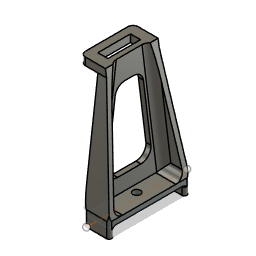
Deckbox_v2_Floor_Assembly (Autodesk Fusion 360 archive; units mm, degrees)
design "DC_DC_Clamp_2_0"
Autodesk Fusion 360 part; units mm, degrees
sketch "Skizze1" plane through (0, 0, 0) normal (0, 0, 1) x (1, 0, 0)
  line L0 (0, 0) -> (0, 46)
  line L1 (0, 46) -> (-7, 46)
  line L2 (-7, 46) -> (-7, 49)
  line L3 (-7, 49) -> (3, 49)
  line L4 (3, 49) -> (3, 2)
  line L5 (3, 2) -> (10, 2)
  line L6 (10, 2) -> (10, 0)
  line L7 (10, 0) -> (0, 0)
  line L8 (3, 49) -> (10, 2)
  dimension "d1" = 46
  dimension "d2" = 3
  dimension "d3" = 7
  dimension "d4" = 10
  dimension "d5" = 2
  dimension "d6" = 3
  constraint coincident L0.start L7.end
  constraint vertical L0
  constraint perpendicular L0 L1
  constraint perpendicular L1 L2
  constraint perpendicular L2 L3
  constraint perpendicular L3 L4
  constraint perpendicular L2 L5
  constraint perpendicular L5 L6
  constraint perpendicular L0 L7
  measures "d1" distance of L0.start L1
  measures "d2" distance of L1.end L2.end
  measures "d3" distance of L0.end L1.end
  measures "d4" distance of L6.end L0.start
  measures "d5" distance of L5 L7
  measures "d6" distance of L0 L4
extrude "Extrusion1" add sketch "Skizze1" along normal mid plane 32
sketch "Skizze2" plane through (0, 49, 0) normal (0, 1, 0) x (-1, 0, 0)
  line L0 (7, -16) -> (7, 16)
  line L1 (7, 16) -> (-3, 16)
  line L2 (-3, -16) -> (7, -16)
  line L3 (36, 0) -> (0, 0) construction
  line L4 (4, -6.5) -> (0, -6.5)
  line L5 (0, -6.5) -> (0, 6.5)
  line L6 (0, 6.5) -> (4, 6.5)
  line L7 (4, 6.5) -> (4, -6.5)
  line L8 (-3, 16) -> (-3, -16)
  dimension "d9" = 13
  dimension "d10" = 4
  constraint coincident L3.end origin
  constraint horizontal L3
  constraint horizontal L4
  constraint vertical L5
  constraint horizontal L6
  constraint vertical L7
  constraint symmetric L3 L4 L6
  constraint coincident L3.end L5
  measures "d9" distance of L4 L6
  measures "d10" distance of L4.start L4.end
extrude "Extrusion2" cut sketch "Skizze2" against normal through all contours L4 L5 L6 L7
sketch "Skizze3" plane through (0, 0, 0) normal (1, 0, 0) x (0, 0, -1)
  line L0 (10.5, 49) -> (-10.5, 49)
  line L1 (-10.5, 49) -> (-10.5, 46)
  line L2 (-10.5, 46) -> (10.5, 46) construction
  line L3 (10.5, 46) -> (10.5, 49)
  line L4 (0, 0) -> (0, 53) construction
  line L5 (16, 0) -> (-16, 0) construction
  line L6 (-16, 0) -> (-16, 2) construction
  line L7 (-16, 2) -> (16, 2) construction
  line L8 (16, 2) -> (16, 0) construction
  line L9 (16, 2) -> (10.5, 46)
  line L10 (-16, 2) -> (-10.5, 46)
  line L11 (16, 46) -> (-16, 46)
  line L12 (16, 49) -> (-16, 49)
  line L13 (16, 0) -> (-16, 0)
  line L14 (16, 0) -> (16, 46)
  line L15 (-16, 46) -> (-16, 0)
  line L16 (16, 2) -> (16, 50)
  line L17 (16, 50) -> (-16, 50)
  line L18 (-16, 50) -> (-16, 2)
  line L19 (0, 8) -> (9.2033, 8)
  line L20 (9.2033, 8) -> (5.2033, 40)
  line L21 (5.2033, 40) -> (0, 40)
  line L22 (-5.2033, 40) -> (0, 40)
  line L23 (-9.2033, 8) -> (-5.2033, 40)
  line L24 (0, 8) -> (-9.2033, 8)
  dimension "d12" = 2
  dimension "d13" = 21
  dimension "d14" = 50
  dimension "d23" = 6
  dimension "d24" = 6
  dimension "d25" = 6
  constraint horizontal L0
  constraint vertical L1
  constraint horizontal L2
  constraint vertical L3
  constraint coincident L4.start origin
  constraint perpendicular L0 L4
  constraint symmetric L1 L3 L4
  constraint horizontal L5
  constraint vertical L6
  constraint horizontal L7
  constraint vertical L8
  constraint collinear L2 L11
  constraint collinear L0 L12
  constraint collinear L5 L13
  constraint collinear L8 L14
  constraint collinear L6 L15
  constraint perpendicular L7 L16
  constraint perpendicular L16 L17
  constraint coincident L4 L19.start
  constraint perpendicular L4 L19
  constraint perpendicular L4 L21
  constraint coincident L4 L21.end
  constraint parallel L9 L20
  constraint symmetric L4 L19.start L24.start
  constraint symmetric L4 L19.end L23.start
  constraint symmetric L4 L20.end L22.start
  constraint symmetric L4 L21.end L22.end
  measures "d12" distance of L5 L7
  measures "d13" distance of L1 L3
  measures "d14" distance of L4.start L17
  measures "d23" distance of L7 L19
  measures "d24" distance of L9 L20
  measures "d25" distance of L2 L21
extrude "Extrusion3" cut sketch "Skizze3" along normal through all and the other way through all contours L3 L11 L12 L16 | L1 L11 L12 L18 | L9 L11 L14 L16 | L10 L11 L15 L18 | L19 L20 L21 L22 L23 L24
sketch "Skizze6" plane through (10, 0, 0) normal (1, 0, 0) x (0, 0, -1)
  line L0 (16, 2) -> (-16, 2)
  line L1 (-16, 2) -> (-16, 0)
  line L2 (-16, 0) -> (16, 0)
  line L3 (16, 0) -> (16, 2)
  line L4 (0, 2) -> (13.9844, 2)
  line L5 (13.9844, 2) -> (8.1094, 49)
  line L6 (8.1094, 49) -> (-0.0505, 49)
  line L7 (-0.0505, 61) -> (-0.0505, 49) construction
  line L8 (0, 2) -> (0, -14) construction
  line L9 (-10.5, 49) -> (10.5, 49)
  line L10 (16, 2) -> (10.5, 46)
  line L11 (-8.2104, 49) -> (-0.0505, 49)
  line L12 (-14.0854, 2) -> (-8.2104, 49)
  line L13 (-0.1009, 2) -> (-14.0854, 2)
  dimension "d20" = 2
  constraint coincident L0 L4.end
  constraint parallel L0 L6
  constraint vertical L7
  constraint coincident L0 L4.start
  constraint collinear L7 L8
  constraint collinear L6 L9
  constraint parallel L5 L10
  constraint coincident origin L8
  constraint symmetric L4.end L7 L12.start
  constraint symmetric L5.end L7 L11.start
  constraint symmetric L6.end L7 L11.end
  constraint symmetric L4.start L7 L13.start
  measures "d20" distance of L5 L10
extrude "Extrusion5" cut sketch "Skizze6" against normal blind 8 contours L0 L4 L5 L6 L9 L11 L12 L13
sketch "Skizze4" plane through (0, 0, 0) normal (0, 1, 0) x (1, 0, 0)
  line L0 (-10, 0) -> (15, 0) construction
  circle A0 centre (5, 0) radius 1.5
  dimension "d16" = 5
  dimension "d17" = 3
  constraint horizontal L0
  constraint coincident L0 A0.centre
  measures "d16" distance of origin A0.centre
  measures "d17" diameter of A0
extrude "Extrusion4" cut sketch "Skizze4" along normal through all
sketch "Skizze7" plane through (0, 0, 0) normal (0, -1, 0) x (1, 0, 0)
  circle A0 centre (5, 0) radius 1.5
  line L0 (10, -16) -> (10, 16)
  line L1 (10, 16) -> (0, 16)
  line L2 (0, 16) -> (0, -16)
  line L3 (0, -16) -> (10, -16)
  line L4 (5, -20) -> (5, 20) construction
  constraint perpendicular L1 L4
fillet "Abrundung1" radius 4 4 edges at (1, 8, -9.2033) (1, 8, 9.2033) (1, 40, -5.2033) (1, 40, 5.2033)
fillet "Abrundung2" radius 3 4 edges at (6, 2, 14.0854) (6, 2, -13.9844) (2, 25.5, 11.1479) (2, 25.5, -11.0469)
fillet "Abrundung3" radius 2 2 edges at (-7, 47.5, -10.5) (-7, 47.5, 10.5)
sketch "Skizze8" plane through (0, 0, 0) normal (0, -1, 0) x (1, 0, 0)
  line L0 (10, 16) -> (0, 16)
  line L1 (0, 16) -> (0, 14)
  line L2 (0, 14) -> (10, 14)
  line L3 (10, 14) -> (10, 16)
  line L4 (10, 16) -> (0, 16)
  line L5 (0, 0) -> (21, 0) construction
  line L6 (5, 0) -> (5, 31) construction
  line L7 (10, -16) -> (10, 16)
  line L8 (0, 16) -> (0, -16)
  line L9 (0, -14) -> (10, -14)
  line L10 (0, -16) -> (0, -14)
  line L11 (10, -16) -> (0, -16)
  line L12 (10, -14) -> (10, -16)
  dimension "d32" = 2
  dimension "d33" = 10
  constraint horizontal L0
  constraint vertical L1
  constraint horizontal L2
  constraint vertical L3
  constraint collinear L0 L4
  constraint coincident L5.start origin
  constraint horizontal L5
  constraint coincident L5 L6.start
  constraint perpendicular L2 L6
  constraint symmetric L1 L3 L6
  constraint symmetric L6 L7 L8
  constraint symmetric L0.start L5 L7.start
  constraint symmetric L0.end L5 L8.end
  constraint symmetric L1.end L5 L9.start
  constraint symmetric L2.end L5 L9.end
  measures "d32" distance of L0 L2
  measures "d33" distance of L1 L3
extrude "Extrusion6" add sketch "Skizze8" along normal blind 4 contours L0 L1 L2 L3 L4 L7 L8 | L7 L8 L9 L10 L11 L12
fillet "Abrundung4" radius 1 10 edges at (10, -2, 14) (10, -1, 16) (0, -1, 16) (0, -2, 14) (10, -2, -14) (0, -2, -14) (0, -1, -16) (10, -1, -16) (5, 0, 14) (5, 0, -14)

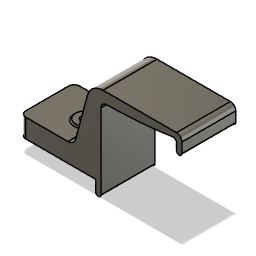
design "Pi_haken_2_0"
Autodesk Fusion 360 part; units mm, degrees
sketch "Skizze1" plane through (0, 0, 0) normal (0, 0, 1) x (1, 0, 0)
  line L0 (-85.7317, 64) -> (69.3607, 64) construction
  line L1 (2, 64) -> (2, 62) construction
  line L2 (2, 62) -> (-37, 62) construction
  arc A0 (3.9784, 62.0107) -> (29, 64) centre (2, 245.25) ccw
  line L3 (29, 64) -> (30, 63.25)
  line L4 (32, 63.25) -> (32, 66)
  line L5 (32, 66) -> (2.7668, 66)
  line L6 (-8, 43) -> (-28, 43)
  line L7 (-28, 43) -> (-28, 41)
  line L8 (2, 41) -> (2, 60.0108)
  line L9 (30, 63.25) -> (30, 59.25)
  line L10 (30, 59.25) -> (32, 59.25)
  line L11 (32, 59.25) -> (32, 63.25)
  line L12 (0, 41) -> (0, 31)
  line L13 (0, 31) -> (2, 31)
  line L14 (2, 31) -> (2, 41)
  line L15 (-95, 41) -> (0, 41) construction
  line L16 (2, 41) -> (26.9938, 41) construction
  line L17 (-28, 41) -> (0, 41)
  line L18 (-8, 43) -> (-3.0288, 61.5529)
  arc A1 (3.9784, 62.0107) -> (2, 60.0108) centre (4, 60.0108) ccw
  arc A2 (2.7668, 66) -> (-3.0288, 61.5529) centre (2.7668, 60) ccw
  line L19 (0, 81.6118) -> (0, 79.7535)
  line L20 (0, 79.7535) -> (0, 12.6342) construction
  point P0 (29, 64)
  dimension "d1" = 64
  dimension "d2" = 41
  dimension "d3" = 2
  dimension "d4" = 2
  dimension "d5" = 27
  dimension "d6" = 1
  dimension "d7" = 4
  dimension "d8" = 2
  dimension "d9" = 2
  dimension "d10" = 10
  dimension "d11" = 28
  dimension "d14" = 2
  dimension "d15" = 6
  dimension "d16" = 15
  dimension "d17" = 10
  dimension "d19" = 2
  constraint horizontal L0
  constraint horizontal L15
  constraint coincident L0 L1.start
  constraint perpendicular L0 L1
  constraint coincident L0 P0
  constraint perpendicular L1 L2
  constraint tangent L2 A0
  constraint coincident P0 A0.end
  constraint perpendicular L4 L5
  constraint coincident L7.end L15
  constraint perpendicular L7 L15
  constraint coincident L8.start L15
  constraint collinear L1 L8
  constraint perpendicular L9 L10
  constraint collinear L4 L11
  constraint vertical L12
  constraint horizontal L13
  constraint vertical L14
  constraint collinear L15 L16
  constraint perpendicular L12 L17
  constraint coincident L1.end L8
  constraint coincident L1.end A0
  constraint tangent L8 A1
  constraint tangent A0 A1
  constraint tangent L18 A2
  constraint tangent L5 A2
  constraint parallel L6 L15
  constraint horizontal L5
  constraint vertical L19
  constraint coincident origin L20
  constraint vertical L20
  constraint collinear L12 L20
  measures "d1" distance of origin L0
  measures "d2" distance of origin L15
  measures "d3" distance of origin L1
  measures "d4" distance of L1.start L1.end
  measures "d5" distance of L1 P0
  measures "d6" horizontal distance of P0 L3.end
  measures "d7" distance of L3.end L9.end
  measures "d8" distance of L9.end L10.end
  measures "d9" distance of P0 L5
  measures "d10" distance of L13 L16
  measures "d11" distance of L7.end L12.start
  measures "d14" radius of A1
  measures "d15" radius of A2
  measures "d16" angle of L8 L18
  measures "d17" distance of L6.start L8
  measures "d19" vertical distance of L6.end L12.start
extrude "Extrusion1" add sketch "Skizze1" along normal mid plane 20
sketch "Skizze2" plane through (0, 0, 0) normal (-1, 0, 0) x (0, 0, 1)
  line L0 (-10, 41) -> (-4.05, 41)
  line L1 (-4.05, 41) -> (-4.05, 36)
  line L2 (-4.05, 36) -> (-10, 36)
  line L3 (-10, 36) -> (-10, 41)
  line L4 (-10, 31) -> (-10, 41)
  line L5 (-10, 41) -> (10, 41)
  line L6 (0, 57.7062) -> (0, 0) construction
  line L7 (10, 36) -> (10, 41)
  line L8 (4.05, 36) -> (10, 36)
  line L9 (4.05, 41) -> (4.05, 36)
  line L10 (10, 41) -> (4.05, 41)
  dimension "d21" = 5.95
  dimension "d22" = 5
  constraint horizontal L0
  constraint vertical L1
  constraint horizontal L2
  constraint vertical L3
  constraint collinear L3 L4
  constraint collinear L0 L5
  constraint vertical L6
  constraint coincident L6.end origin
  constraint symmetric L0.start L6 L5.end
  constraint symmetric L0.end L6 L9.start
  constraint symmetric L1.end L6 L8.start
  constraint symmetric L2.end L6 L7.start
  measures "d21" distance of L1.end L2.end
  measures "d22" distance of L0 L2
extrude "Extrusion2" add sketch "Skizze2" along normal blind 28
sketch "Skizze3" plane through (0, 41, 0) normal (0, -1, 0) x (1, 0, 0)
  line L0 (-28, -4.05) -> (0, -4.05)
  line L1 (0, -4.05) -> (0, 4.05)
  line L2 (0, 4.05) -> (-28, 4.05)
  line L3 (-28, 4.05) -> (-28, -4.05)
  circle A0 centre (-14, 0) radius 1.5
  line L4 (-14, -41.0811) -> (-14, 36.0811) construction
  line L5 (-28, -10) -> (-28, -4.05)
  line L6 (0, -10) -> (0, 10)
  line L7 (34, 0) -> (-40, 0) construction
  dimension "d25" = 3
  constraint vertical L4
  constraint coincident A0.centre L4
  constraint perpendicular L4 L7
  constraint coincident A0.centre L7
  measures "d25" diameter of A0
extrude "Extrusion3" cut sketch "Skizze3" against normal through all contours A0
sketch "Skizze4" plane through (0, 43, 0) normal (0, 1, 0) x (-1, 0, 0)
  circle A0 centre (14, 0) radius 1.5
  line L0 (28, -10) -> (28, 10)
  line L1 (28, 10) -> (8, 10)
  line L2 (8, 10) -> (8, -10)
  line L3 (8, -10) -> (28, -10)
  circle A1 centre (14, 0) radius 3.5
  circle A2 centre (14, 0) radius 1.5
  dimension "d27" = 7
  constraint concentric A0 A1
  constraint concentric A1 A2
  measures "d27" diameter of A1
extrude "Extrusion4" add sketch "Skizze4" along normal blind 0.5 contours A1
fillet "Abrundung6" radius 2 2 edges at (-28, 39.5, 10) (-28, 39.5, -10)
fillet "Abrundung1" radius 3 1 edges at (-8, 43, 0)
fillet "Abrundung2" radius 2 1 edges at (32, 66, 0)
fillet "Abrundung3" radius 1 4 edges at (0, 31, 0) (2, 31, 0) (-14, 36, 4.05) (-14, 36, -4.05)
fillet "Abrundung4" radius 1 2 edges at (32, 59.25, 0) (30, 59.25, 0)
chamfer "Fase1" distance 0.5 angle 45 1 edges at (-10.7369, 43, 1.2657)

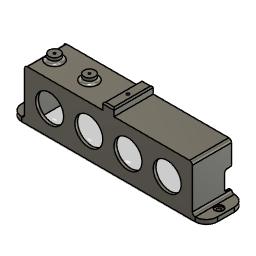
design "AC_DC_housing_v2"
Autodesk Fusion 360 part; units mm, degrees
sketch "Skizze1" plane through (0, 0, 0) normal (0, 0, 1) x (1, 0, 0)
  line L0 (0, 0) -> (-70, 0)
  line L1 (-70, 0) -> (-70, 3)
  line L2 (-60, 3) -> (-70, 3)
  line L3 (-60, 3) -> (-60, 36)
  line L4 (-60, 36) -> (0, 36)
  line L5 (0, 130) -> (0, 0) construction
  line L6 (60, 36) -> (0, 36)
  line L7 (0, 0) -> (70, 0)
  line L8 (60, 3) -> (60, 36)
  line L9 (70, 0) -> (70, 3)
  line L10 (60, 3) -> (70, 3)
  dimension "d1" = 36
  dimension "d2" = 120
  dimension "d3" = 10
  dimension "d4" = 3
  constraint coincident L0.start L5.end
  constraint horizontal L0
  constraint perpendicular L0 L1
  constraint perpendicular L1 L2
  constraint perpendicular L2 L3
  constraint perpendicular L3 L4
  constraint perpendicular L0 L5
  constraint symmetric L0.start L5 L7.start
  constraint symmetric L0.end L5 L7.end
  constraint symmetric L1.end L5 L9.end
  constraint symmetric L2.start L5 L8.start
  constraint symmetric L3.end L5 L6.start
  constraint symmetric L4.end L5 L6.end
  measures "d1" distance of L0 L4
  measures "d2" distance of L3 L8
  measures "d3" distance of L1.end L2.start
  measures "d4" distance of L2 L0.start
extrude "Extrusion1" add sketch "Skizze1" along normal blind 28
sketch "Skizze2" plane through (0, 0, 0) normal (1, 0, 0) x (0, 0, -1)
  line L0 (0, 0) -> (0, 34.419)
  line L1 (0, 34.419) -> (-26, 33.2838)
  line L2 (-26, 33.2838) -> (-26, 0.2838)
  line L3 (-26, 0.2838) -> (-19.5, 0)
  line L4 (-19.5, 0) -> (0, 0)
  line L5 (-1.75, 0) -> (-22.5, 0)
  line L6 (-19.5, 0) -> (-26, 0)
  line L7 (-26, 0.2838) -> (-26, 0)
  dimension "d7" = 2.5
  dimension "d8" = 2.5
  dimension "d9" = 33
  dimension "d10" = 6.5
  dimension "d11" = 26
  constraint coincident L0.start L4.end
  constraint vertical L0
  constraint parallel L0 L2
  constraint parallel L4 L5
  constraint parallel L5 L6
  constraint perpendicular L6 L7
  measures "d7" angle of L3 L4
  measures "d8" angle of L1 L4
  measures "d9" distance of L1.end L2.end
  measures "d10" distance of L2 L3.end
  measures "d11" distance of L0 L2
extrude "Extrusion2" cut sketch "Skizze2" along normal mid plane 118
chamfer "Fase1" distance 26 angle 2.5 2 edges at (59, 16.6419, 26) (-59, 16.6419, 26) measured on face at (59, 22.5676, 8.6667) measured on face at (-59, 22.5676, 8.6667)
sketch "Skizze3" plane through (-60, 0, 0) normal (-1, 0, 0) x (0, 0, 1)
  line L0 (0, 36) -> (0, 3)
  line L1 (0, 3) -> (28, 3)
  line L2 (28, 3) -> (28, 36)
  line L3 (28, 36) -> (0, 36)
  line L4 (0, 27.419) -> (3, 27.419)
  line L5 (5, 25.419) -> (5, 15.419)
  line L6 (3, 13.419) -> (0, 13.419)
  line L7 (0, 13.419) -> (0, 27.419)
  arc A0 (5, 25.419) -> (3, 27.419) centre (3, 25.419) ccw
  arc A1 (3, 13.419) -> (5, 15.419) centre (3, 15.419) ccw
  point P0 (5, 27.419)
  point P1 (5, 13.419)
  point P2 (0, 34.419)
  dimension "d16" = 14
  dimension "d17" = 5
  dimension "d18" = 7
  dimension "d19" = 2
  constraint horizontal L4
  constraint vertical L5
  constraint horizontal L6
  constraint vertical L7
  constraint coincident L0 L4.start
  constraint coincident P0 L5
  constraint coincident P0 L4
  constraint tangent L5 A0
  constraint tangent L4 A0
  constraint coincident P1 L5
  constraint coincident P1 L6
  constraint tangent L5 A1
  constraint tangent L6 A1
  constraint equal A0 A1
  measures "d16" distance of P0 P1
  measures "d17" distance of P1 L6.end
  measures "d18" distance of L4.start P2
  measures "d19" radius of A0
extrude "Extrusion3" cut sketch "Skizze3" against normal blind 5 contours L0 L4 L5 L6 L7 A0 A1
sketch "Skizze4" plane through (60, 0, 0) normal (1, 0, 0) x (0, 0, -1)
  line L0 (0, 3) -> (0, 36)
  line L1 (0, 36) -> (-28, 36)
  line L2 (-28, 36) -> (-28, 3)
  line L3 (-28, 3) -> (0, 3)
  line L4 (0, 19.419) -> (-3, 19.419)
  line L5 (-5, 17.419) -> (-5, 7.419)
  line L6 (-3, 5.419) -> (0, 5.419)
  line L7 (0, 5.419) -> (0, 19.419)
  arc A0 (-3, 19.419) -> (-5, 17.419) centre (-3, 17.419) ccw
  arc A1 (-5, 7.419) -> (-3, 5.419) centre (-3, 7.419) ccw
  point P0 (-5, 19.419)
  point P1 (-5, 5.419)
  point P2 (0, 34.419)
  dimension "d23" = 14
  dimension "d25" = 5
  dimension "d26" = 2
  constraint horizontal L4
  constraint vertical L5
  constraint horizontal L6
  constraint vertical L7
  constraint coincident L0 L4.start
  constraint coincident P0 L5
  constraint coincident P0 L4
  constraint tangent L5 A0
  constraint tangent L4 A0
  constraint coincident P1 L5
  constraint coincident P1 L6
  constraint tangent L5 A1
  constraint tangent L6 A1
  constraint equal A0 A1
  measures "d23" distance of P0 P1
  measures "d25" distance of L5 L7
  measures "d26" radius of A0
extrude "Extrusion4" cut sketch "Skizze4" against normal blind 5 contours L0 L4 L5 L6 L7 A0 A1
fillet "Abrundung3" radius 2 2 edges at (57.8648, 16.6419, 26) (-57.8648, 16.6419, 26)
fillet "Abrundung4" radius 2 9 edges at (58.4742, 33.8931, 12.0436) (57.3333, 33.308, 25.4447) (0, 33.2838, 26) (-57.3333, 33.308, 25.4447) (-58.4742, 33.8931, 12.0436) (60, 3, 14) (-60, 3, 14) (60, 36, 14) (-60, 36, 14)
fillet "Abrundung5" radius 8 4 edges at (70, 1.5, 28) (70, 1.5, 0) (-70, 1.5, 0) (-70, 1.5, 28)
sketch "Skizze5" plane through (0, 0, 0) normal (0, -1, 0) x (1, 0, 0)
  arc A0 (-62, 28) -> (-70, 20) centre (-62, 20) ccw
  line L0 (-70, 20) -> (-70, 8)
  arc A1 (-70, 8) -> (-62, 0) centre (-62, 8) ccw
  line L1 (-62, 0) -> (-59, 0)
  line L2 (-59, 0) -> (-57.9483, 24.0872)
  arc A2 (-55.9502, 26) -> (-57.9483, 24.0872) centre (-55.9502, 24) ccw
  line L3 (-55.9502, 26) -> (55.9502, 26)
  arc A3 (57.9483, 24.0872) -> (55.9502, 26) centre (55.9502, 24) ccw
  line L4 (57.9483, 24.0872) -> (59, 0)
  line L5 (59, 0) -> (62, 0)
  arc A4 (62, 0) -> (70, 8) centre (62, 8) ccw
  line L6 (70, 8) -> (70, 20)
  arc A5 (70, 20) -> (62, 28) centre (62, 20) ccw
  line L7 (62, 28) -> (-62, 28)
  line L8 (98.5458, 14) -> (-90, 14) construction
  line L9 (1.75, 0) -> (22.5, 0)
  circle A6 centre (65, 14) radius 1.5
  line L10 (0, -42.6314) -> (0, 44.2372) construction
  line L11 (0, -42.6314) -> (0, 44.2372) construction
  circle A7 centre (-65, 14) radius 1.5
  dimension "d40" = 3
  dimension "d41" = 5
  constraint perpendicular L0 L8
  constraint coincident L8 A6.centre
  constraint coincident origin L10
  constraint vertical L10
  constraint symmetric A6 L10 A7
  constraint symmetric L11.start L10 L10.start
  constraint symmetric L11.end L10 L10.end
  measures "d40" diameter of A6
  measures "d41" distance of L6 A6.centre
extrude "Extrusion5" cut sketch "Skizze5" along normal through all and the other way through all contours A6 | A7
fillet "Abrundung6" radius 1 4 edges at (59.5, 5.419, 0) (59.5, 19.419, 0) (-59.5, 27.419, 0) (-59.5, 13.419, 0)
sketch "Skizze6" plane through (0, 3, 0) normal (0, 1, 0) x (-1, 0, 0)
  circle A0 centre (-65, 14) radius 1.5
  arc A1 (-70, 8) -> (-62, 0) centre (-62, 8) ccw
  line L0 (-62, 0) -> (-62, 28)
  arc A2 (-62, 28) -> (-70, 20) centre (-62, 20) ccw
  line L1 (-70, 20) -> (-70, 8)
  circle A3 centre (65, 14) radius 3
  circle A4 centre (65, 14) radius 1.5
  circle A5 centre (-65, 14) radius 3
  dimension "d45" = 6
  constraint concentric A3 A4
  constraint concentric A0 A5
  constraint equal A3 A5
  measures "d45" diameter of A3
extrude "Extrusion6" cut sketch "Skizze6" against normal blind 1 contours A5 | A3
sketch "Skizze7" plane through (0, 36, 0) normal (0, 1, 0) x (-1, 0, 0)
  line L0 (58, 0) -> (58, 28)
  line L1 (58, 28) -> (-58, 28)
  line L2 (-58, 28) -> (-58, 0)
  line L3 (-58, 0) -> (58, 0)
  circle A0 centre (52.5, 14) radius 4
  circle A1 centre (52.5, 14) radius 0.75
  line L4 (-66.9318, 14) -> (75.9318, 14) construction
  line L5 (23, 27) -> (57, 27) construction
  line L6 (57, 27) -> (57, 1) construction
  line L7 (57, 1) -> (23, 1) construction
  line L8 (23, 1) -> (23, 27) construction
  line L9 (40, 39) -> (40, -17) construction
  circle A2 centre (27.5, 14) radius 4
  circle A3 centre (27.5, 14) radius 0.75
  line L10 (0, 20) -> (0, 2.5)
  dimension "d48" = 26
  dimension "d49" = 34
  dimension "d50" = 25
  dimension "d51" = 8
  dimension "d52" = 1.5
  dimension "d53" = 40
  constraint concentric A0 A1
  constraint horizontal L4
  constraint symmetric L1 L3 L4
  constraint horizontal L5
  constraint vertical L6
  constraint horizontal L7
  constraint vertical L8
  constraint symmetric L4 L5 L7
  constraint vertical L9
  constraint symmetric L6 L8 L9
  constraint symmetric A0 L9 A2
  constraint symmetric A1 L9 A3
  measures "d48" distance of L5 L7
  measures "d49" distance of L5.start L5.end
  measures "d50" distance of A0.centre A2.centre
  measures "d51" diameter of A0
  measures "d52" diameter of A1
  measures "d53" distance of L9 L10
extrude "Extrusion7" add sketch "Skizze7" along normal blind 4 contours A0 | A2
fillet "Abrundung7" radius 2 2 edges at (-23.7707, 36, 15.4465) (-48.7707, 36, 15.4465)
sketch "Skizze9" plane through (0, 0, 0) normal (0, -1, 0) x (1, 0, 0)
  circle A0 centre (65, 14) radius 1.5
  circle A1 centre (-65, 14) radius 1.5
  arc A2 (-62, 28) -> (-70, 20) centre (-62, 20) ccw
  line L0 (-70, 20) -> (-70, 8)
  arc A3 (-70, 8) -> (-62, 0) centre (-62, 8) ccw
  line L1 (-62, 0) -> (-59, 0)
  line L2 (-59, 0) -> (-57.9483, 24.0872)
  arc A4 (-55.9502, 26) -> (-57.9483, 24.0872) centre (-55.9502, 24) ccw
  line L3 (-55.9502, 26) -> (55.9502, 26)
  arc A5 (57.9483, 24.0872) -> (55.9502, 26) centre (55.9502, 24) ccw
  line L4 (57.9483, 24.0872) -> (59, 0)
  arc A6 (62, 0) -> (70, 8) centre (62, 8) ccw
  line L5 (70, 8) -> (70, 20)
  arc A7 (70, 20) -> (62, 28) centre (62, 20) ccw
  line L6 (62, 28) -> (-62, 28)
  line L7 (59, 0) -> (60, 0)
  line L8 (59, 0) -> (58.105, 20.5)
  line L9 (60, 20.5) -> (60, 0)
  line L10 (60, 20.5) -> (58.105, 20.5)
  line L11 (0, -13) -> (0, 43) construction
  line L12 (-59, 0) -> (-58.105, 20.5)
  line L13 (-60, 20.5) -> (-58.105, 20.5)
  line L14 (-60, 20.5) -> (-60, 0)
  line L15 (-59, 0) -> (-60, 0)
  dimension "d60" = 1
  dimension "d61" = 7.5
  constraint coincident L4.end L7.start
  constraint coincident L4 L8.end
  constraint horizontal L10
  constraint perpendicular L10 L11
  constraint symmetric L4.end L11 L1.end
  constraint symmetric L8.end L11 L12.end
  constraint symmetric L9.start L11 L13.start
  constraint symmetric L7.end L11 L14.end
  measures "d60" distance of L4.end L7.end
  measures "d61" distance of L6 L10
extrude "Extrusion9" add sketch "Skizze9" along normal blind 1 contours L1 L2 L12 L13 L14 L15 | L4 L7 L8 L9 L10
sketch "Skizze10" plane through (0, 0, 0) normal (1, 0, 0) x (0, 0, -1)
  line L0 (19.6814, 0) -> (-52, 0) construction
  line L1 (-21.4519, 0) -> (0, -0.9366)
  line L2 (0, -0.9366) -> (-21.4519, -0.9366) construction
  line L3 (-21.4519, 0) -> (-21.4519, -0.9366) construction
  line L4 (0, 7.8481) -> (0, -14.5746) construction
  line L5 (-10, -0.9366) -> (-10, -0.5) construction
  line L6 (-28, 5) -> (-28, 34)
  line L7 (-21.4519, 0) -> (-26, 0)
  line L8 (-26, 0) -> (-26, -3)
  line L9 (-26, -3) -> (0, -3.3632)
  line L10 (0, -0.9366) -> (0, -3.3632)
  dimension "d64" = 2.5
  dimension "d65" = 0.5
  dimension "d66" = 18
  dimension "d67" = 26
  dimension "d68" = 3
  constraint horizontal L0
  constraint coincident L0 L1.start
  constraint parallel L0 L2
  constraint perpendicular L2 L3
  constraint coincident origin L4
  constraint vertical L4
  constraint coincident L1.end L4
  constraint coincident L2 L5.start
  constraint perpendicular L0 L5
  constraint coincident L1 L5.end
  constraint coincident origin L0
  constraint coincident L0 L7.end
  constraint perpendicular L7 L8
  constraint midpoint L4 L9.end
  measures "d64" angle of L0 L1
  measures "d65" distance of L0 L5.end
  measures "d66" distance of L5 L6
  measures "d67" horizontal distance of L8.end L9.end
  measures "d68" distance of L7.end L8.end
extrude "Extrusion10" cut sketch "Skizze10" along normal through all and the other way through all
sketch "Skizze11" plane through (0, 36, 0) normal (0, 1, 0) x (-1, 0, 0)
  line L0 (-4, 0) -> (-4, 28)
  line L1 (4, 28) -> (4, 0)
  line L2 (0, 20) -> (0, 2.5)
  circle A0 centre (0, 14) radius 1
  line L3 (-58, 0) -> (58, 0)
  line L4 (58, 28) -> (-58, 28)
  line L5 (4, 0) -> (-4, 0)
  line L6 (4, 28) -> (-4, 28)
  dimension "d70" = 8
  dimension "d71" = 2
  constraint vertical L0
  constraint vertical L1
  constraint symmetric L0 L1 L2
  constraint perpendicular L0 L6
  measures "d70" distance of L0 L1
  measures "d71" diameter of A0
extrude "Extrusion11" add sketch "Skizze11" along normal blind 5
fillet "Abrundung9" radius 1 4 edges at (-4, 41, 14) (0, 41, 0) (4, 41, 14) (0, 41, 28)
sketch "Skizze12" plane through (0, 0, 28) normal (0, 0, 1) x (1, 0, 0)
  line L0 (4, 40) -> (-4, 40)
  line L1 (-4, 40) -> (-4, 36)
  line L2 (-4, 36) -> (-58, 36)
  arc A0 (-58, 36) -> (-60, 34) centre (-58, 34) ccw
  line L3 (-60, 34) -> (-60, 5)
  arc A1 (-62, 3) -> (-60, 5) centre (-62, 5) ccw
  line L4 (-62, 3) -> (-62, 0)
  line L5 (-62, 0) -> (62, 0)
  line L6 (62, 0) -> (62, 3)
  arc A2 (60, 5) -> (62, 3) centre (62, 5) ccw
  line L7 (60, 5) -> (60, 34)
  arc A3 (60, 34) -> (58, 36) centre (58, 34) ccw
  line L8 (58, 36) -> (4, 36)
  line L9 (4, 36) -> (4, 40)
  line L10 (0, 45) -> (0, 0) construction
  line L11 (-77.0065, 18) -> (78.0065, 18) construction
  line L12 (-58, 36) -> (58, 36)
  circle A4 centre (-42, 18) radius 10
  circle A5 centre (-14, 18) radius 10
  circle A6 centre (14, 18) radius 10
  circle A7 centre (42, 18) radius 10
  dimension "d80" = 20
  dimension "d81" = 28
  dimension "d82" = 84
  constraint coincident L10.end origin
  constraint perpendicular L5 L10
  constraint horizontal L11
  constraint coincident L11 A4.centre
  constraint coincident L11 A5.centre
  constraint coincident L11 A6.centre
  constraint coincident L11 A7.centre
  constraint equal A4 A5
  constraint equal A4 A6
  constraint equal A4 A7
  constraint symmetric L10 A5.centre A6.centre
  constraint symmetric L10 A4.centre A7.centre
  measures "d80" diameter of A4
  measures "d81" distance of A5.centre A6.centre
  measures "d82" distance of A4.centre A7.centre
extrude "Extrusion12" cut sketch "Skizze12" along normal through all and the other way through all contours A4 | A5 | A6 | A7
sketch "Skizze13" plane through (0, 36, 0) normal (0, 1, 0) x (-1, 0, 0)
  circle A0 centre (-45, 14) radius 5
  circle A1 centre (-29, 14) radius 5
  line L0 (-37, 40.4914) -> (-37, -23.5086) construction
  line L1 (-60, 28) -> (-60, 0)
  line L2 (0, 20) -> (0, 2.5)
  line L3 (-66.9318, 14) -> (75.9318, 14)
  dimension "d84" = 16
  dimension "d85" = 10
  dimension "d86" = 23
  constraint vertical L0
  constraint equal A0 A1
  constraint symmetric A0.centre A1.centre L0
  constraint coincident A0.centre L3
  measures "d84" distance of A0.centre A1.centre
  measures "d85" diameter of A0
  measures "d86" distance of L0 L1
extrude "Extrusion13" [suppressed]
sketch "Skizze8" plane through (0, 40, 0) normal (0, 1, 0) x (-1, 0, 0)
  circle A0 centre (27.5, 14) radius 0.75
  circle A1 centre (27.5, 14) radius 4
  circle A2 centre (27.5, 14) radius 0.75
  circle A3 centre (52.5, 14) radius 0.75
  circle A4 centre (52.5, 14) radius 0.75
  circle A5 centre (0, 14) radius 1
  circle A6 centre (0, 14) radius 1
  constraint concentric A0 A2
  constraint equal A0 A2
  constraint equal A3 A4
  constraint concentric A3 A4
  constraint tangent A5 A6
  constraint concentric A5 A6
extrude "Extrusion8" cut sketch "Skizze8" along normal through all and the other way through all contours A0 A2 | A3 A4 | A5 A6
